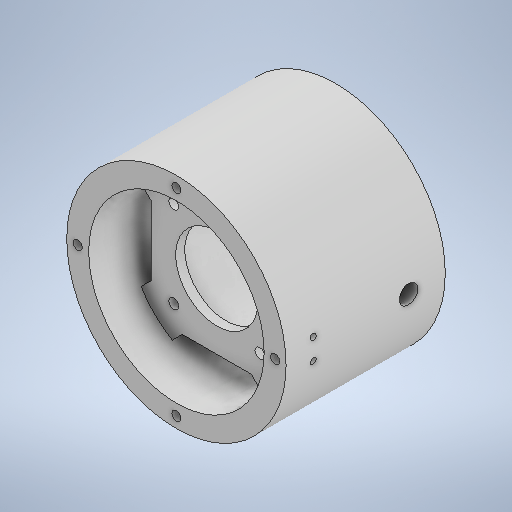
# Autodesk Inventor part: j1 57 mount
Saved by Autodesk Inventor 2025 (Build 290162000, 162)
## iProperties
Created: 2025-07-04
Part Number: j1 57 mount
Material: 一般
Document SubType Name: Modeling
Designer: gavin
Density: 1 g/cm^3
Appearance: 預設
Author: gavin
Autodesk Inventor part; units mm, degrees
sketch "草圖1" plane through (0, 0, 0) normal (0, 0, 1) x (1, 0, 0)
  circle A0 centre (0, 0) radius 60
  circle A1 centre (0, 0) radius 48
  dimension "d0" = 120
  dimension "d1" = 96
  constraints: 2 centre point, 2 coincident
  measures "d0" diameter of A0
  measures "d1" diameter of A1
extrude "擠出1" add sketch "草圖1" along normal blind 27.1 and the other way blind 60
sketch "草圖2" plane through (0, 0, 27.1) normal (0, 0, 1) x (1, 0, 0)
  circle A0 centre (0, 0) radius 54 construction
  circle A1 centre (0, 54) radius 2.5
  circle A2 centre (-54, 0) radius 2.5
  circle A3 centre (0, -54) radius 2.5
  circle A4 centre (54, 0) radius 2.5
  dimension "d6" = 108
  dimension "d7" = 5
  dimension "d10" = 360
  constraints: 4 centre point, 1 coincident, 1 vertical alignment, 11 other
  measures "d7" diameter of A1
extrude "擠出2" cut sketch "草圖2" against normal blind 20
ref_plane "工作平面1" through (0, 0, 0) normal (0, 0, 1) x (1, 0, 0)
sketch "草圖3" plane through (0, 0, 0) normal (0, 0, 1) x (1, 0, 0)
  circle A0 centre (-23.57, 23.57) radius 2.3 projected
  circle A1 centre (23.57, 23.57) radius 2.3 projected
  circle A2 centre (23.57, -23.57) radius 2.3 projected
  circle A3 centre (-23.57, -23.57) radius 2.3 projected
  circle A4 centre (-23.57, 23.57) radius 2.7
  circle A5 centre (23.57, 23.57) radius 2.7
  circle A6 centre (23.57, -23.57) radius 2.7
  circle A7 centre (-23.57, -23.57) radius 2.7
  circle A8 centre (0, 0) radius 22.5
  line L0 (-21.9436, 4.973) -> (-41.3486, 24.3781)
  circle A9 centre (0, 0) radius 48 projected
  line L1 (-24.3781, 41.3486) -> (-4.973, 21.9436)
  line L2 (-23.57, 23.57) -> (0, 0) construction
  circle A10 centre (0, 0) radius 40.5
  line L3 (-41.3486, -24.3781) -> (-21.9436, -4.973)
  line L4 (-4.973, -21.9436) -> (-24.3781, -41.3486)
  line L5 (24.3781, -41.3486) -> (4.973, -21.9436)
  line L6 (21.9436, -4.973) -> (41.3486, -24.3781)
  line L7 (41.3486, 24.3781) -> (21.9436, 4.973)
  line L8 (4.973, 21.9436) -> (24.3781, 41.3486)
  point P0 (-18.8666, 35.8372)
  point P1 (-35.8372, 18.8666)
  point P2 (-35.8372, -18.8666)
  point P3 (-24.3781, -41.3486)
  point P4 (-18.8666, -35.8372)
  point P5 (18.8666, -35.8372)
  point P6 (24.3781, -41.3486)
  point P7 (41.3486, -24.3781)
  point P8 (35.8372, -18.8666)
  point P9 (35.8372, 18.8666)
  point P10 (41.3486, 24.3781)
  point P11 (24.3781, 41.3486)
  point P12 (18.8666, 35.8372)
  dimension "d14" = 5.4
  dimension "d15" = 5.4
  dimension "d16" = 5.4
  dimension "d17" = 5.4
  dimension "d18" = 45
  dimension "d19" = 24
  dimension "d20" = 12
  dimension "d21" = 18
  dimension "d24" = 360
  constraints: 18 end point, 6 centre point, 4 point on circle, 2 coincident, 2 parallel, 25 other
  measures "d14" diameter of A4
  measures "d15" diameter of A5
  measures "d16" diameter of A6
  measures "d17" diameter of A7
  measures "d18" diameter of A8
  measures "d19" distance between parallel lines of L1 L0
  measures "d20" distance from line of A0.centre L1
  measures "d21" radial gap between concentric circles of A8 A10
extrude "擠出3" add sketch "草圖3" along normal blind 5 contours A8 L7 A10 L6 | A8 L8 A10 L7 | L6 A10 L5 A8 | A8 L1 A10 L8 | A10 L8 A9 L7 | L5 A10 L4 A8 | L6 A9 L5 A10 | A8 L0 A10 L1 | L4 A10 L3 A8 | A8 L3 A10 L0 | A10 L0 A9 L1 | L4 A9 L3 A10
sketch "草圖4" plane through (0, 0, -60) normal (0, 0, -1) x (-1, 0, 0)
  circle A0 centre (0, 0) radius 54 construction
  circle A1 centre (0, -54) radius 2.5
  circle A2 centre (46.7654, -27) radius 2.5
  circle A3 centre (46.7654, 27) radius 2.5
  circle A4 centre (0, 54) radius 2.5
  circle A5 centre (-46.7654, 27) radius 2.5
  circle A6 centre (-46.7654, -27) radius 2.5
  dimension "d29" = 108
  dimension "d32" = 360
  dimension "d62" = 5
  constraints: 7 centre point, 2 coincident, 13 other
  measures "d29" diameter of A0
  measures "d62" diameter of A1
extrude "擠出4" cut sketch "草圖4" against normal blind 20
ref_plane "工作平面2" through (28.2, -16.65, -54) normal (1, 0, 0) x (0, 1, 0)
sketch "草圖5" plane through (28.2, -16.65, -54) normal (1, 0, 0) x (0, 1, 0)
  circle A0 centre (16.65, 14) radius 5
  line L0 (-43.35, -6) -> (76.65, -6) projected
  point P0 (16.65, 54)
  dimension "d36" = 10
  dimension "d37" = 20
  constraints: 1 centre point
  measures "d36" diameter of A0
  measures "d37" distance from line of L0 A0.centre
extrude "擠出5" cut sketch "草圖5" along normal through all
ref_plane "工作平面3" through (48, 0, 0) normal (1, 0, 0) x (0, 1, 0)
sketch "草圖7" plane through (48, 0, 0) normal (1, 0, 0) x (0, 1, 0)
  line L0 (9, 15.1) -> (-9, 15.1)
  line L1 (-9, 15.1) -> (-9, 8.85)
  line L2 (-9, 8.85) -> (9, 8.85)
  line L3 (9, 8.85) -> (9, 15.1)
  line L4 (-48, 27.1) -> (48, 27.1) projected
  point P0 (0, 0)
  dimension "d45" = 18
  dimension "d46" = 9
  dimension "d47" = 6.25
  dimension "d48" = 12
  constraints: 8 end point, 2 parallel, 1 horizontal, 1 perpendicular
  measures "d45" distance of L2.end L1.end
  measures "d46" distance from line of point (0, 0) L1
  measures "d47" distance of L2.end L0.start
  measures "d48" distance between parallel lines of L0 L4
extrude "擠出6" add sketch "草圖7" against normal blind 0.85
sketch "草圖8" plane through (47.15, 0, 0) normal (-1, 0, 0) x (0, 0, 1)
  line L0 (15.1, -8.9932) -> (8.85, -8.9932) projected
  line L1 (15.1, -8.9932) -> (15.1, 8.9932) projected
  line L2 (8.85, 8.9932) -> (15.1, 8.9932) projected
  line L3 (8.85, 8.9932) -> (8.85, -8.9932) projected
  line L4 (15.1, 0) -> (8.85, 0)
  circle A0 centre (11.975, 5.75) radius 1.6
  circle A1 centre (11.975, -5.75) radius 1.6
  point P0 (0, 0)
  point P1 (11.975, 8.9932)
  dimension "d52" = 3.2
  dimension "d53" = 5.75
  constraints: 3 midpoint, 2 centre point, 2 end point, 1 symmetric about line, 1 vertical alignment, 1 other
  measures "d52" diameter of A0
  measures "d53" distance from line of L4 A0.centre
extrude "擠出7" cut sketch "草圖8" against normal through all contours A0 | A1
sketch "草圖9" plane through (0, 0, 5) normal (0, 0, 1) x (1, 0, 0)
  line L0 (-24.3781, -41.3486) -> (-18.8666, -35.8372) projected
  arc A0 (-18.8666, -35.8372) -> (18.8666, -35.8372) centre (0, 0) ccw projected
  line L1 (18.8666, -35.8372) -> (24.3781, -41.3486) projected
  line L2 (41.3486, -24.3781) -> (35.8372, -18.8666) projected
  arc A1 (35.8372, -18.8666) -> (35.8372, 18.8666) centre (0, 0) ccw projected
  line L3 (35.8372, 18.8666) -> (41.3486, 24.3781) projected
  line L4 (24.3781, 41.3486) -> (18.8666, 35.8372) projected
  arc A2 (18.8666, 35.8372) -> (-18.8666, 35.8372) centre (0, 0) ccw projected
  line L5 (-18.8666, 35.8372) -> (-24.3781, 41.3486) projected
  line L6 (-41.3486, 24.3781) -> (-35.8372, 18.8666) projected
  arc A3 (-35.8372, 18.8666) -> (-35.8372, -18.8666) centre (0, 0) ccw projected
  line L7 (-35.8372, -18.8666) -> (-41.3486, -24.3781) projected
  circle A4 centre (23.57, -23.57) radius 2.7 projected
  circle A5 centre (23.57, 23.57) radius 2.7 projected
  circle A6 centre (-23.57, 23.57) radius 2.7 projected
  circle A7 centre (-23.57, -23.57) radius 2.7 projected
  circle A8 centre (0, 0) radius 22.5 projected
  line L8 (18.8666, -35.8372) -> (-18.8666, -35.8372)
  line L9 (35.8372, 18.8666) -> (35.8372, -18.8666)
  line L10 (-18.8666, 35.8372) -> (18.8666, 35.8372)
  line L11 (-35.8372, -18.8666) -> (-35.8372, 18.8666)
  arc A9 (-24.3781, 41.3486) -> (-41.3486, 24.3781) centre (0, 0) ccw projected
  arc A10 (-41.3486, -24.3781) -> (-24.3781, -41.3486) centre (0, 0) ccw projected
  arc A11 (24.3781, -41.3486) -> (41.3486, -24.3781) centre (0, 0) ccw projected
  arc A12 (41.3486, 24.3781) -> (24.3781, 41.3486) centre (0, 0) ccw projected
  point P0 (35.8372, 18.8666)
  point P1 (-18.8666, 35.8372)
  point P2 (-35.8372, -18.8666)
  dimension "d58" = 360
  constraints: 8 end point, 1 horizontal, 13 other
extrude "擠出8" cut sketch "草圖9" against normal up to surface (5 mm away) contours L8 A0 | A3 L11 | L9 A1 | A2 L10
thread "螺紋1" size "M5x0.8" class "6H" standard "ANSI Metric M Profile" full length
thread "螺紋2" size "M5x0.8" class "6H" standard "ANSI Metric M Profile" full length
thread "螺紋3" size "M5x0.8" class "6H" standard "ANSI Metric M Profile" full length
thread "螺紋4" size "M5x0.8" class "6H" standard "ANSI Metric M Profile" full length
thread "螺紋5" size "M5x0.8" class "6H" standard "ANSI Metric M Profile" full length
thread "螺紋6" size "M5x0.8" class "6H" standard "ANSI Metric M Profile" full length
thread "螺紋7" size "M5x0.8" class "6H" standard "ANSI Metric M Profile" full length
thread "螺紋8" size "M5x0.8" class "6H" standard "ANSI Metric M Profile" full length
thread "螺紋9" size "M5x0.8" class "6H" standard "ANSI Metric M Profile" full length
thread "螺紋10" size "M5x0.8" class "6H" standard "ANSI Metric M Profile" full length
equation "\"d20\" = 0.5 * d19"
equation "\"d46\" = 0.5 * d45"
